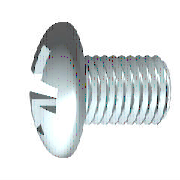
# Autodesk Inventor part: EN ISO 7045 - M3 x 10 - 4.8 - H
Saved by Autodesk Inventor 2024 (Build 280153000, 153)
## iProperties
IsCustomPart: 0
Created: 2023-01-19
Part Number: EN ISO 7045 - M3 x 10 - 4.8 - H
Material: Stainless Steel, 440C
Description: Pan head with type H or type Z cross recess. Product grade A
Document SubType Name: Modeling
Standard: EN ISO 7045
Designer: alexz
Standards Organization: BSI
Language: en-US
Size Designation: M3 x 10 - 4.8 - H
Categories: <MemberInstance><Categories><Category DisplayName="Fasteners" InternalName="e4da775c-781d-43d5-af7c-5136215cf5a6" Mnemonic="FSTN"><Category DisplayName="Bolts" InternalName="536e6df0-f778-49ac-b2f2-25c71d2aa0b2" Mnemonic="SCRW"><CategoryParameter DisplayName="Nominal Diameter Designation" InternalName="03caf894-eafd-4c09-a035-916ac084b87b" Mnemonic="nomdiadesig"/><CategoryParameter DisplayName="Nominal Length" InternalName="238ecbaf-3e6c-45dd-aa95-4068c8e0fd02" Mnemonic="nomlen"/><CategoryParameter DisplayName="Thread Designation" InternalName="586d5e89-370a-4089-914f-0110033585c7" Mnemonic="thrdesign"/><CategoryParameter DisplayName="Thread Series Designation" InternalName="87c5849c-b3a5-4c3e-9c9b-2feecef9be86" Mnemonic="thrserdsgn"/><CategoryParameter DisplayName="Nominal Diameter" InternalName="8bbe3f8e-44cf-40a9-a251-3a6edc8168d6" Mnemonic="nomdia"/><CategoryParameter DisplayName="Thread Type" InternalName="b4bbb7bc-d6aa-4c9f-a9a9-4152b9f6fe49" Mnemonic="thrtype"/><CategoryParameter DisplayName="Thread Pitch" InternalName="bb82302e-82d8-4176-8fc1-c5d7bb17d5ad" Mnemonic="pitch1"/><CategoryParameter DisplayName="Threads per Unit" InternalName="bdc6e7d2-ffd0-4d9c-a173-16b95ebb912d" Mnemonic="thrperunit1"/><CategoryParameter DisplayName="Thread Class" InternalName="ebc0d23b-2cc6-4d2a-b376-d52aae53bab6" Mnemonic="thrclss"/><Category DisplayName="Round Head" InternalName="df3578aa-538f-4805-96a8-2439eb0c3cf7" Mnemonic="RNDSCRW"><CategoryParameter DisplayName="Grip Length" InternalName="2c6ace26-543b-4217-91c4-9cdf8c3ec6f1" Mnemonic="grplen"/><CategoryParameter DisplayName="Head Height" InternalName="2d152238-84fe-49ae-94c3-3fee884c292b" Mnemonic="headh"/><CategoryParameter DisplayName="Property Class" InternalName="85496db6-1567-48ed-b0d4-aa1f03366005" Mnemonic="propclss"/><CategoryParameter DisplayName="Thread Length" InternalName="a1e5edc5-4ca7-4847-8786-65b14d35af16" Mnemonic="thrlen"/><CategoryParameter DisplayName="Shank Diameter" InternalName="c22f1a48-b8d5-43ef-ac5e-546ba91c0bd6" Mnemonic="grpdia"/><CategoryParameter DisplayName="Head Diameter" InternalName="e71ee7a1-06fd-425c-ba3b-09769885677c" Mnemonic="headdia"/></Category></Category></Category><Category DisplayName="DataType" InternalName="23b78d0f-2648-40c6-8793-ca6db495c9e8" Mnemonic="DATATYPE"><CategoryParameter DisplayName="DisplayName" InternalName="05415f3d-3907-474b-a020-eb9d644f4cf3" Mnemonic="DISPLAYNAME"/><CategoryParameter DisplayName="Standard" InternalName="0c0a119c-1e12-4c84-803f-101930972f5e" Mnemonic="STANDARD"/><CategoryParameter DisplayName="Description" InternalName="13903e3d-64b1-4950-80da-f627842ea37f" Mnemonic="DESCRIPTION"/><CategoryParameter DisplayName="Designation" InternalName="2675968c-4ce5-49e0-a4f5-552d29089031" Mnemonic="DESIGNATION"/><CategoryParameter DisplayName="Default Row" InternalName="2af9ec52-faaa-4026-b378-f9fa4afca842" Mnemonic="DEFAULTROW"/><CategoryParameter DisplayName="Folder Name" InternalName="3f06958e-8713-4116-9be7-ed6184ecc97b" Mnemonic="FOLDERNAME"/><CategoryParameter DisplayName="Revision Guid" InternalName="45a75005-10b1-4dfc-8d6d-dfe629f0b93c" Mnemonic="REVISIONGUID"/><CategoryParameter DisplayName="FileName" InternalName="8b46a4cc-9585-4fed-90c3-899f57e09a73" Mnemonic="FILENAME"/><CategoryParameter DisplayName="StdsOrg" InternalName="8f5914e1-4693-403f-8ab5-d37768198c9d" Mnemonic="STDSORG"/><CategoryParameter DisplayName="Family Version" InternalName="914462f6-6e19-4b14-ba84-155b9680b1d0" Mnemonic="FAMILYREVISION"/><CategoryParameter DisplayName="Standard Revision" InternalName="91d5a463-65c2-4fde-b823-3b7fea5e8e17" Mnemonic="STANDARDREVISION"/><CategoryParameter DisplayName="Member Revision" InternalName="a65d44b9-392f-4f4f-857b-e4b3d54996fe" Mnemonic="MEMBERREVISION"/><CategoryParameter DisplayName="ClipFormat" InternalName="bc51e27b-3422-4e78-93ef-cec197ddf230" Mnemonic="CLIPFORMAT"/><CategoryParameter DisplayName="Manufacturer" InternalName="cd6c7a72-a28a-4e50-99a9-2c7f4e13e5ad" Mnemonic="MANUFACTURER"/><CategoryParameter DisplayName="InternalName" InternalName="cf1d0246-76d9-4b4a-8305-fa0409afb5c1" Mnemonic="INTERNALNAME"/><CategoryParameter DisplayName="IsMetric" InternalName="e2385c5b-1ea4-4823-96a8-8de651266ec3" Mnemonic="ISMETRIC"/><Category DisplayName="Part" InternalName="c0e0b642-3bcb-4cc8-9e80-f96d35c4afa4" Mnemonic="PART"><CategoryParameter DisplayName="Part Number" InternalName="016b6077-bfbe-49bd-92c9-d8d59c39c941" Mnemonic="PARTNUMBER"/><CategoryParameter DisplayName="Stock Number" InternalName="4dba7c1c-e26c-444e-836c-b08b433409a8" Mnemonic="STOCKNUMBER"/><CategoryParameter DisplayName="Material Key" InternalName="5c9a8adb-dd2b-4535-b97f-0a94a95fe41f" Mnemonic="MATERIALKEY"/><CategoryParameter DisplayName="Material" InternalName="818a152a-d3c3-49ca-80ee-df7d91421b8e" Mnemonic="MATERIAL"/></Category></Category><Category DisplayName="Legacy Map DA" InternalName="924fff40-ddd0-4eff-ad42-30e3774ef79e" Mnemonic="LEGACYMAPDA"><CategoryParameter DisplayName="DACookie" InternalName="316934ee-8fe1-4c7a-9c36-f2d79e1add1a" Mnemonic="DACOOKIE"/></Category><Category DisplayName="LegacyMap" InternalName="cd87c42b-3e48-431e-b5c0-1cbeb14dfe77" Mnemonic="LEGACYMAP"><CategoryParameter DisplayName="unique DA member ID" InternalName="0918ad47-427f-4fed-ae26-24c81c58f590" Mnemonic="DACOOKIE"/><CategoryParameter DisplayName="Merge11 ID" InternalName="0ee8fb18-e2ed-4f39-96f6-1f4b5f50aa71" Mnemonic="MERGE11"/><CategoryParameter DisplayName="unique CC member ID" InternalName="5193edd4-b2b0-4ab4-9d54-de900eee34e0" Mnemonic="CCCOOKIE"/><CategoryParameter DisplayName="Split ID" InternalName="72b5c83c-be7f-45c4-ae51-9160ea6deb26" Mnemonic="SPLIT"/><CategoryParameter DisplayName="MemberID" InternalName="8e5e0294-fc51-4c8f-b3d7-003dc5ed94f6" Mnemonic="MEMBERID"/><CategoryParameter DisplayName="CatalogName" InternalName="d99d1e27-aa94-4de2-af4c-c348882a6f4f" Mnemonic="CATALOGNAME"/><CategoryParameter DisplayName="FamilyNumber" InternalName="e705e1f4-09cb-413e-91f9-551b4188271e" Mnemonic="FAMILYNUMBER"/></Category></Categories><FamilyTemplate Id="si0151"><FamilyTemplateParameters><FamilyTemplateParameter ObjectType="kUserParameterObject" ValueType="xs:double" Id="1" ObjectReferenceKey="GUL"/><FamilyTemplateParameter ObjectType="kUserParameterObject" ValueType="xs:double" Id="2" ObjectReferenceKey="SPD"/><FamilyTemplateParameter ObjectType="kUserParameterObject" ValueType="xs:double" Id="3" ObjectReferenceKey="NLG"/><FamilyTemplateParameter ObjectType="kUserParameterObject" ValueType="xs:double" Id="4" ObjectReferenceKey="KOD"/><FamilyTemplateParameter ObjectType="kUserParameterObject" ValueType="xs:double" Id="5" ObjectReferenceKey="SBR"/><FamilyTemplateParameter ObjectType="kUserParameterObject" ValueType="xs:double" Id="6" ObjectReferenceKey="KR"/><FamilyTemplateParameter ObjectType="kUserParameterObject" ValueType="xs:double" Id="7" ObjectReferenceKey="PTC"/><FamilyTemplateParameter ObjectType="kUserParameterObject" ValueType="xs:double" Id="8" ObjectReferenceKey="GEL"/><FamilyTemplateParameter ObjectType="kUserParameterObject" ValueType="xs:double" Id="9" ObjectReferenceKey="THREADDIA"/><FamilyTemplateParameter ObjectType="kUserParameterObject" ValueType="xs:double" Id="10" ObjectReferenceKey="TOA"/><FamilyTemplateParameter ObjectType="kUserParameterObject" ValueType="xs:double" Id="11" ObjectReferenceKey="BDM"/><FamilyTemplateParameter ObjectType="kUserParameterObject" ValueType="xs:double" Id="12" ObjectReferenceKey="RR"/><FamilyTemplateParameter ObjectType="kUserParameterObject" ValueType="xs:double" Id="13" ObjectReferenceKey="STI"/><FamilyTemplateParameter ObjectType="kUserParameterObject" ValueType="xs:double" Id="14" ObjectReferenceKey="TPU"/><FamilyTemplateParameter ObjectType="kUserParameterObject" ValueType="xs:double" Id="15" ObjectReferenceKey="KOH"/><FamilyTemplateParameter ObjectType="kUserParameterObject" ValueType="xs:double" Id="16" ObjectReferenceKey="SDM"/><FamilyTemplateParameter ObjectType="kUserParameterObject" ValueType="xs:double" Id="17" ObjectReferenceKey="NND"/><FamilyTemplateParameter ObjectType="kUserParameterObject" ValueType="xs:double" Id="18" ObjectReferenceKey="GD"/><FamilyTemplateParameter ObjectType="kUserParameterObject" ValueType="xs:double" Id="19" ObjectReferenceKey="GAL"/><FamilyTemplateParameter ObjectType="kUserParameterObject" ValueType="xs:double" Id="20" ObjectReferenceKey="KEWI"/><FamilyTemplateParameter ObjectType="kUserParameterObject" ValueType="xs:double" Id="21" ObjectReferenceKey="GD1"/><FamilyTemplateParameter ObjectType="kPropertyObject" ValueType="xs:string" Id="100" ObjectReferenceKey="{32853F0F-3444-11d1-9E93-0060B03C1CA6}" SubObjectId="52"/><FamilyTemplateParameter ObjectType="kPropertyObject" ValueType="xs:string" Id="105" ObjectReferenceKey="{32853F0F-3444-11d1-9E93-0060B03C1CA6}" SubObjectId="5"/><FamilyTemplateParameter ObjectType="kPartComponentDefinitionObject" ValueType="xs:string" Id="110" SubObjectId="Material"/><FamilyTemplateParameter ObjectType="kThreadFeatureObject" ValueType="xs:structure" Id="300" ObjectReferenceKey="1002000010000000aa0f0000000000008000000000000000" SubObjectId="ThreadInfo"><FamilyTemplateParameter ObjectType="" ValueType="xs:string" Id="301" SubObjectId="ThreadDesignation"/><FamilyTemplateParameter ObjectType="" ValueType="xs:string" Id="302" SubObjectId="ThreadType"/><FamilyTemplateParameter ObjectType="" ValueType="xs:string" Id="303" SubObjectId="ThreadClass"/></FamilyTemplateParameter></FamilyTemplateParameters></FamilyTemplate><CategoryParameterMap><ParamToTemplateMap><ParamToTemplate CategoryParameter="//CategoryParameter[@InternalName='05415f3d-3907-474b-a020-eb9d644f4cf3']" ConstantValue="BS EN ISO 7045 H - Metric"/><ParamToTemplate CategoryParameter="//CategoryParameter[@InternalName='cf1d0246-76d9-4b4a-8305-fa0409afb5c1']" ConstantValue="e59574d2-6d1d-4d5b-84ae-6524854ac01c"/><ParamToTemplate CategoryParameter="//CategoryParameter[@InternalName='3f06958e-8713-4116-9be7-ed6184ecc97b']" ConstantValue="BS EN ISO 7045 H"/><ParamToTemplate CategoryParameter="//CategoryParameter[@InternalName='914462f6-6e19-4b14-ba84-155b9680b1d0']" ConstantValue="10"/><ParamToTemplate CategoryParameter="//CategoryParameter[@InternalName='bc51e27b-3422-4e78-93ef-cec197ddf230']" ConstantValue="CF_INVENTOR.STDPARTS"/><ParamToTemplate CategoryParameter="//CategoryParameter[@InternalName='e2385c5b-1ea4-4823-96a8-8de651266ec3']" ConstantValue="true"/><ParamToTemplate CategoryParameter="//CategoryParameter[@InternalName='13903e3d-64b1-4950-80da-f627842ea37f']" ConstantValue="Pan head with type H or type Z cross recess. Product grade A"/><ParamToTemplate CategoryParameter="//CategoryParameter[@InternalName='8f5914e1-4693-403f-8ab5-d37768198c9d']" ConstantValue="BSI"/><ParamToTemplate CategoryParameter="//CategoryParameter[@InternalName='0c0a119c-1e12-4c84-803f-101930972f5e']" ConstantValue="EN ISO 7045"/><ParamToTemplate CategoryParameter="//CategoryParameter[@InternalName='cd6c7a72-a28a-4e50-99a9-2c7f4e13e5ad']" TemplateParameter="104"/><ParamToTemplate CategoryParameter="//CategoryParameter[@InternalName='91d5a463-65c2-4fde-b823-3b7fea5e8e17']" TemplateParameter="103"/><ParamToTemplate CategoryParameter="//CategoryParameter[@InternalName='45a75005-10b1-4dfc-8d6d-dfe629f0b93c']" ConstantValue="3a716aec-bc6d-4ddc-afff-2484deaed6d0"/><ParamToTemplate CategoryParameter="//CategoryParameter[@InternalName='2af9ec52-faaa-4026-b378-f9fa4afca842']" ConstantValue="1"/><ParamToTemplate CategoryParameter="//CategoryParameter[@InternalName='d99d1e27-aa94-4de2-af4c-c348882a6f4f']" ConstantValue="BSI"/><ParamToTemplate CategoryParameter="//CategoryParameter[@InternalName='e705e1f4-09cb-413e-91f9-551b4188271e']" ConstantValue="17"/><ParamToTemplate CategoryParameter="//CategoryParameter[@InternalName='8b46a4cc-9585-4fed-90c3-899f57e09a73']" ConstantValue="EN ISO 7045 - M3 x 10 - 4.8 - H(1)"/><ParamToTemplate CategoryParameter="//CategoryParameter[@InternalName='a65d44b9-392f-4f4f-857b-e4b3d54996fe']" ConstantValue="128F147A-D3FA-4472-BBD4-866B856F0525"/><ParamToTemplate CategoryParameter="//CategoryParameter[@InternalName='2c6ace26-543b-4217-91c4-9cdf8c3ec6f1']" ConstantValue="1"/><ParamToTemplate CategoryParameter="//CategoryParameter[@InternalName='ebc0d23b-2cc6-4d2a-b376-d52aae53bab6']" ConstantValue="6g"/><ParamToTemplate CategoryParameter="//CategoryParameter[@InternalName='03caf894-eafd-4c09-a035-916ac084b87b']" ConstantValue="M3"/><ParamToTemplate CategoryParameter="//CategoryParameter[@InternalName='b4bbb7bc-d6aa-4c9f-a9a9-4152b9f6fe49']" ConstantValue="ISO Metric profile"/><ParamToTemplate CategoryParameter="//CategoryParameter[@InternalName='8e5e0294-fc51-4c8f-b3d7-003dc5ed94f6']" ConstantValue="35"/><ParamToTemplate CategoryParameter="//CategoryParameter[@InternalName='316934ee-8fe1-4c7a-9c36-f2d79e1add1a']" ConstantValue="*Bsi~I7045H~M3x10 - 4.8 - H~10*"/><ParamToTemplate CategoryParameter="//CategoryParameter[@InternalName='c22f1a48-b8d5-43ef-ac5e-546ba91c0bd6']" TemplateParameter="11"/><ParamToTemplate CategoryParameter="//CategoryParameter[@InternalName='2675968c-4ce5-49e0-a4f5-552d29089031']" TemplateParameter="100"/><ParamToTemplate CategoryParameter="//CategoryParameter[@InternalName='a1e5edc5-4ca7-4847-8786-65b14d35af16']" TemplateParameter="8"/><ParamToTemplate CategoryParameter="//CategoryParameter[@InternalName='e71ee7a1-06fd-425c-ba3b-09769885677c']" TemplateParameter="4"/><ParamToTemplate CategoryParameter="//CategoryParameter[@InternalName='2d152238-84fe-49ae-94c3-3fee884c292b']" TemplateParameter="15"/><ParamToTemplate CategoryParameter="//CategoryParameter[@InternalName='818a152a-d3c3-49ca-80ee-df7d91421b8e']" TemplateParameter="110"/><ParamToTemplate CategoryParameter="//CategoryParameter[@InternalName='238ecbaf-3e6c-45dd-aa95-4068c8e0fd02']" TemplateParameter="3"/><ParamToTemplate CategoryParameter="//CategoryParameter[@InternalName='8bbe3f8e-44cf-40a9-a251-3a6edc8168d6']" TemplateParameter="17"/><ParamToTemplate CategoryParameter="//CategoryParameter[@InternalName='016b6077-bfbe-49bd-92c9-d8d59c39c941']" TemplateParameter="105"/><ParamToTemplate CategoryParameter="//CategoryParameter[@InternalName='bb82302e-82d8-4176-8fc1-c5d7bb17d5ad']" TemplateParameter="7"/><ParamToTemplate CategoryParameter="//CategoryParameter[@InternalName='586d5e89-370a-4089-914f-0110033585c7']" TemplateParameter="301"/><ParamToTemplate CategoryParameter="//CategoryParameter[@InternalName='bdc6e7d2-ffd0-4d9c-a173-16b95ebb912d']" TemplateParameter="14"/></ParamToTemplateMap></CategoryParameterMap></MemberInstance>
Density: 7.75 g/cm^3
Appearance: Semi-Polished
Author: alexz
Autodesk Inventor part; units mm, degrees
ref_plane "YZ Plane" through (0, 0, 0) normal (1, 0, 0) x (0, 1, 0)
sketch "Sketch1" plane through (0, 0, 0) normal (0, 0, 1) x (1, 0, 0)
  line L0 (10, 0) -> (10, 1.5)
  line L1 (10, 1.5) -> (1, 1.5)
  line L2 (3.9624, 5.08) -> (3.9624, 5.08)
  arc A0 (-1.5792, 2.7449) -> (-2.4, 0) centre (2.6, 0) ccw
  line L3 (-2.4, 0) -> (-2.4, 2.7162)
  line L4 (-2.1999, 1.4002) -> (-1.036, 0.8199)
  line L5 (-1.036, 0.8199) -> (-0.6, 0)
  line L6 (-0.6, 0) -> (10, 0)
  line L7 (-5.121, 0) -> (12.5202, 0) projected
  line L8 (0, -1.016) -> (0, 6.096) projected
  line L9 (-2.1999, 1.4002) -> (-2.4, 1.5) construction
  line L10 (-1.5792, 2.7449) -> (-2.4, 2.7162)
  line L11 (-1.5792, 2.7449) -> (0, 2.8)
  line L12 (0, 2.8) -> (0, 1.3647)
  line L13 (0, 1.3647) -> (0.6933, 1.3647)
  line L14 (0.6933, 1.3647) -> (1, 1.5)
  line L15 (1, 1.5) -> (0, 1.5) construction
  dimension "d1" = 3
  dimension "d2" = 1.8
  dimension "d11" = 3
  dimension "d12" = 62
  dimension "d13" = 26.5
  dimension "d17" = 5.6
  dimension "d19" = 2
  dimension "d20" = 2.4
  dimension "d21" = 5
  dimension "d23" = 2.7294
  dimension "d24" = 9
  dimension "d25" = 0.3067
  dimension "d28" = 10
  constraints: 28 end point, 5 point on line, 4 collinear, 4 point on circle, 3 parallel, 2 perpendicular, 1 centre point, 1 horizontal, 1 tangent
  measures "d1" diameter of L1 L6
  measures "d2" distance from line of L5.end L3
  measures "d11" diameter of L9.end L6
  measures "d12" angle of L5 L6
  measures "d13" angle of L4 L6
  measures "d17" diameter of L11.end L6
  measures "d19" angle of L11 L6
  measures "d20" distance between parallel lines of L3 L12
  measures "d21" radius of A0
  measures "d23" diameter of L13 L6
  measures "d24" distance of L0.end L1.end
  measures "d25" horizontal distance of L13.end L1.end
  measures "d28" distance between parallel lines of L0 L12
revolve "Body" add sketch "Sketch1" angle 360 about axis through (-0.6, 0, 0) along (1, 0, 0) contours L6 L8 L13 L14 L1 L0 | L6 L5 L4 A0 L11 L8
ref_plane "Work Plane1" through (-2.4, 0, 0) normal (1, 0, 0) x (0, 1, 0)
sketch "Sketch2" plane through (-2.4, 0, 0) normal (1, 0, 0) x (0, 1, 0)
  circle A0 centre (0, 0) radius 2.7449 projected
  line L0 (-3.8428, 0) -> (3.8428, 0) projected
  line L1 (0, -3.8428) -> (0, 3.8428) projected
  line L2 (0, 1.5) -> (0, 0) construction
  line L3 (0, 0) -> (1.5, 0) construction
  arc A1 (0.45, 0) -> (0, 0.45) centre (0, 0) ccw construction
  line L4 (0, 0) -> (1.9409, 1.9409) construction
  line L5 (0.215, 1.4845) -> (0.257, 0.4578)
  line L6 (1.4845, 0.215) -> (0.4578, 0.257)
  arc A2 (1.5, 0) -> (1.4845, 0.215) centre (0, 0) ccw
  arc A3 (0.215, 1.4845) -> (0, 1.5) centre (0, 0) ccw
  arc A4 (1.4845, 0.215) -> (0.215, 1.4845) centre (0, 0) ccw
  arc A5 (1.4845, -0.215) -> (1.5, 0) centre (0, 0) ccw
  arc A6 (0, -1.5) -> (0.215, -1.4845) centre (0, 0) ccw
  arc A7 (0.215, -1.4845) -> (1.4845, -0.215) centre (0, 0) ccw
  arc A8 (-1.4845, 0.215) -> (-1.5, 0) centre (0, 0) ccw
  arc A9 (0, 1.5) -> (-0.215, 1.4845) centre (0, 0) ccw
  arc A10 (-0.215, 1.4845) -> (-1.4845, 0.215) centre (0, 0) ccw
  arc A11 (-0.215, -1.4845) -> (0, -1.5) centre (0, 0) ccw
  arc A12 (-1.4845, -0.215) -> (-0.215, -1.4845) centre (0, 0) ccw
  arc A13 (-1.5, 0) -> (-1.4845, -0.215) centre (0, 0) ccw
  arc A14 (0.525, 0) -> (0, 0.525) centre (0, 0) ccw construction
  arc A15 (0.257, 0.4578) -> (0.4578, 0.257) centre (0.4664, 0.4664) ccw
  line L7 (0.215, -1.4845) -> (0.257, -0.4578)
  line L8 (1.4845, -0.215) -> (0.4578, -0.257)
  arc A16 (0.4578, -0.257) -> (0.257, -0.4578) centre (0.4664, -0.4664) ccw
  line L9 (-0.215, 1.4845) -> (-0.257, 0.4578)
  line L10 (-1.4845, 0.215) -> (-0.4578, 0.257)
  arc A17 (-0.4578, 0.257) -> (-0.257, 0.4578) centre (-0.4664, 0.4664) ccw
  line L11 (-0.215, -1.4845) -> (-0.257, -0.4578)
  arc A18 (-0.257, -0.4578) -> (-0.4578, -0.257) centre (-0.4664, -0.4664) ccw
  line L12 (-1.4845, -0.215) -> (-0.4578, -0.257)
  dimension "d4" = 45
  dimension "d5" = 0.9
  dimension "d6" = 3
  dimension "d7" = 0.215
  dimension "d14" = 1.05
  constraints: 38 point on circle, 22 end point, 19 symmetric about line, 18 centre point, 4 coincident, 3 collinear, 3 point on line, 3 tangent, 1 perpendicular, 21 other
  measures "d4" angle of L4 L3
  measures "d5" diameter of A1
  measures "d6" diameter of A4
  measures "d7" distance from line of L5.start L2
  measures "d14" diameter of A14
extrude "Slot" add sketch "Sketch2" along normal up to next draft 5 contours L6 A15 L5 A4 | A7 L7 A16 L8 | L9 A17 L10 A10 | A12 L12 A18 L11
revolve "Cut" cut sketch "Sketch1" angle 360 about axis through (-10, 0, 0) along (1, 0, 0) contours L3 L10 A0
fillet "Fillet1" radius 1 1 edges at (-1.5792, -2.7449, 0)
fillet "Fillet2" radius 0.086 7 edges at (-2.1999, 0, 1.4002) (-2.1999, 0.9901, 0.9901) (-2.1999, 0, -1.4002) (-2.1999, -1.4002, 0) (-2.1999, 0.9901, -0.9901) (-2.1999, -0.9901, 0.9901) (-2.1999, -0.9901, -0.9901)
thread "Thread" size "M3x0.5" class "6g" standard "ISO Metric profile" length 9
chamfer "Chamfer1" distance 0.3067 distance2 0.3068 1 edges at (10, -1.5, 0) measured on face at (10, -0.1088, 0.5667)
ref_plane "Work Plane3" through (3.4925, 0, 0) normal (0, 1, 0) x (1, 0, 0)
equation "\"d5\" = 0.3 * SDM"
equation "\"d6\" = SDM"
equation "\"d7\" = 0.5 * SBR"
equation "\"d14\" = 0.35 * SDM"
equation "\"d1\" = GD"
equation "\"d2\" = STI"
equation "\"d11\" = SDM"
equation "\"d17\" = KOD"
equation "\"d19\" = KEWI"
equation "\"d20\" = KOH"
equation "\"d21\" = KR"
equation "\"d23\" = BDM"
equation "\"d24\" = GEL"
equation "\"d25\" = GAL"
equation "\"d28\" = NLG"
equation "\"d29\" = RR"
equation "\"d16\" = 0.2 * SBR"
equation "\"d8\" = GEL"
equation "\"d26\" = -0.5 * SPD + 0.5 * GD"
equation "\"GD\" = 3"
equation "\"NLG\" = 10"
equation "\"GEL\" = 9"
equation "\"KOD\" = 5.6"
equation "\"KOH\" = 2.4"
equation "\"SDM\" = 3"
equation "\"STI\" = 1.8"
equation "\"SBR\" = 0.43"
equation "\"GAL\" = 0.61345 * PTC"
equation "\"SPD\" = NND - 1.2269 * PTC"
equation "\"KEWI\" = 2deg"
equation "\"d3\" = -KOH"
equation "\"KR\" = 5"
equation "\"BDM\" = 2.72937"
equation "\"GUL\" = 0.61345 * PTC"
equation "\"RR\" = 1"
equation "\"PTC\" = 0.5"
equation "\"THREADDIA\" = 3"
equation "\"TOA\" = 30deg"
equation "\"NND\" = 3"
equation "\"GD1\" = THREADDIA - 1.2269 * PTC"
body "Solid1"
